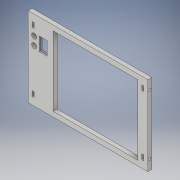
# Autodesk Inventor part: Topshelf
Saved by Autodesk Inventor 2019 (Build 230136000, 136)
## iProperties
Created: 2018-12-26
Part Number: Topshelf
Material: Generic
Document SubType Name: Modeling
Designer: Martin
Density: 1 g/cm^3
Appearance: Default
Author: Martin
Autodesk Inventor part; units mm, degrees
ref_plane "YZ Plane" through (0, 0, 0) normal (1, 0, 0) x (0, 1, 0)
ref_plane "XZ Plane" through (0, 0, 0) normal (0, 1, 0) x (-1, 0, 0)
ref_plane "XY Plane" through (0, 0, 0) normal (0, 0, 1) x (1, 0, 0)
sketch "Sketch1" plane through (0, 0, 0) normal (0, 0, 1) x (1, 0, 0)
  line L0 (-59.525, 40) -> (60.475, 40)
  line L1 (60.475, 40) -> (60.475, -40)
  line L2 (60.475, -40) -> (-59.525, -40)
  line L3 (-59.525, -40) -> (-59.525, 40)
  line L4 (-59.525, 40) -> (60.475, -40) construction
  line L5 (60.475, 40) -> (-59.525, -40) construction
  line L6 (-34.525, -65) -> (-34.525, 60.8703) construction
  line L7 (50.475, -61.0061) -> (50.475, 64.8642) construction
  line L8 (-67.2304, -35) -> (77.4738, -35) construction
  line L9 (-68.2264, 35) -> (76.4779, 35) construction
  line L10 (-2.025, -66.0646) -> (-2.025, 59.8057) construction
  line L11 (2.975, -64.9269) -> (2.975, 60.9434) construction
  line L12 (-67.6256, -30) -> (77.0786, -30) construction
  line L13 (-69.0671, 30) -> (75.6371, 30) construction
  line L14 (55.475, -60.5874) -> (55.475, 65.2829) construction
  line L15 (-54.525, -62.7211) -> (-54.525, 63.1492) construction
  line L16 (-55.475, -32.5) -> (-53.575, -32.5)
  line L17 (-53.575, -32.5) -> (-53.575, -27.5)
  line L18 (-53.575, -27.5) -> (-55.475, -27.5)
  line L19 (-55.475, -27.5) -> (-55.475, -32.5)
  line L20 (-55.475, -32.5) -> (-53.575, -27.5) construction
  line L21 (-53.575, -32.5) -> (-55.475, -27.5) construction
  line L22 (56.425, -32.5) -> (54.525, -32.5)
  line L23 (54.525, -32.5) -> (54.525, -27.5)
  line L24 (54.525, -27.5) -> (56.425, -27.5)
  line L25 (56.425, -27.5) -> (56.425, -32.5)
  line L26 (56.425, -32.5) -> (54.525, -27.5) construction
  line L27 (54.525, -32.5) -> (56.425, -27.5) construction
  line L28 (-53.575, 32.5) -> (-55.475, 32.5)
  line L29 (-55.475, 32.5) -> (-55.475, 27.5)
  line L30 (-55.475, 27.5) -> (-53.575, 27.5)
  line L31 (-53.575, 27.5) -> (-53.575, 32.5)
  line L32 (-53.575, 32.5) -> (-55.475, 27.5) construction
  line L33 (-55.475, 32.5) -> (-53.575, 27.5) construction
  line L34 (56.425, 32.5) -> (54.525, 32.5)
  line L35 (54.525, 32.5) -> (54.525, 27.5)
  line L36 (54.525, 27.5) -> (56.425, 27.5)
  line L37 (56.425, 27.5) -> (56.425, 32.5)
  line L38 (56.425, 32.5) -> (54.525, 27.5) construction
  line L39 (54.525, 32.5) -> (56.425, 27.5) construction
  line L40 (-34.525, 35) -> (50.475, 35)
  line L41 (50.475, 35) -> (50.475, -35)
  line L42 (50.475, -35) -> (-34.525, -35)
  line L43 (-34.525, -35) -> (-34.525, 35)
  point P0 (0.475, 0)
  point P1 (-2.025, 35)
  point P2 (2.975, -35)
  point P3 (50.475, 35)
  point P4 (55.475, 36)
  point P5 (56, 37)
  point P6 (-54.525, -30)
  point P7 (55.475, -30)
  point P8 (-54.525, 30)
  point P9 (55.475, 30)
  dimension "d0" = 120
  dimension "d1" = 80
  dimension "d9" = 25
  dimension "d10" = 10
  dimension "d11" = 5
  dimension "d12" = 5
  dimension "d20" = 10
  dimension "d21" = 10
  dimension "d22" = 5
  dimension "d23" = 5
  dimension "d26" = 1.9
  dimension "d27" = 5
  dimension "d28" = 1.9
  dimension "d29" = 1.9
  dimension "d30" = 5
  dimension "d31" = 1.9
  constraints: 88 end point, 23 point on line, 12 parallel, 10 horizontal, 9 midpoint, 6 perpendicular, 6 vertical
  measures "d0" distance of L1.end L2.end
  measures "d1" distance of L0.end L1.end
  measures "d9" distance between parallel lines of L6 L3
  measures "d10" distance between parallel lines of L1 L7
  measures "d11" distance between parallel lines of L8 L2
  measures "d12" distance between parallel lines of L0 L9
  measures "d20" distance between parallel lines of L12 L2
  measures "d21" distance between parallel lines of L13 L0
  measures "d22" distance between parallel lines of L14 L1
  measures "d23" distance between parallel lines of L15 L3
  measures "d26" distance of L18.end L17.end
  measures "d27" distance of L17.end L16.end
  measures "d28" distance of L23.end L24.end
  measures "d29" distance of L30.end L29.end
  measures "d30" distance of L29.end L28.end
  measures "d31" distance of L36.end L35.end
extrude "Extrusion1" add sketch "Sketch1" along normal blind 4 contours L0 L1 L2 L3 | L19 L18 L17 L16 | L22 L23 L24 L25 | L31 L30 L29 L28 | L37 L36 L35 L34 | L40 L41 L42 L43
sketch "Sketch2" plane through (60.475, -40, 0) normal (1, 0, 0) x (0, 0, -1)
  line L0 (0, 40) -> (-8.8455, 40) construction
  line L1 (-2, -5.0193) -> (-2, 56.2537) construction
  line L2 (-4, 0) -> (-4, 80) construction
  line L3 (1.2244, 10) -> (-7.6211, 10) construction
  line L4 (0, 0) -> (-4, 0) construction
  circle A0 centre (-2, 10) radius 1.25
  circle A1 centre (-2, 70) radius 1.25
  dimension "d4" = 2
  dimension "d5" = 10
  dimension "d6" = 2.5
  constraints: 6 end point, 2 centre point, 2 horizontal, 2 point on line, 1 symmetric about line, 1 vertical, 1 other
  measures "d4" distance between parallel lines of L1 L2
  measures "d5" distance between parallel lines of L3 L4
  measures "d6" diameter of A0
extrude "Extrusion3" cut sketch "Sketch2" against normal blind 10
extrude "Extrusion4" cut sketch "Sketch1" along normal blind 10 contours L19 L18 L17 L16 | L22 L23 L24 L25 | L31 L30 L29 L28 | L37 L36 L35 L34
ref_plane "Work Plane1" through (0.475, -40, 0) normal (1, 0, 0) x (0, 0, -1)
mirror "Mirror1" about plane through (0.475, -40, 0) normal (1, 0, 0) of "Extrusion3"
extrude "Extrusion6" cut sketch "Sketch1" along normal blind 10 contours L40 L41 L42 L43
sketch "Sketch3" plane through (0, 0, 4) normal (0, 0, 1) x (1, 0, 0)
  line L0 (0, 0) -> (-78.4813, 0) construction
  line L1 (-44.525, 48.1643) -> (-44.525, -53.6198) construction
  line L2 (-34.525, -35) -> (-34.525, 35) construction
  line L3 (-48.525, 23.5) -> (-40.525, 23.5)
  line L4 (-40.525, 23.5) -> (-40.525, 10)
  line L5 (-40.525, 10) -> (-48.525, 10)
  line L6 (-48.525, 10) -> (-48.525, 23.5)
  line L7 (-53.525, 48.2216) -> (-53.525, -53.5625) construction
  circle A0 centre (-53.525, 20.95) radius 2.55
  circle A1 centre (-53.525, 12.55) radius 2.55
  line L8 (-47.3423, 23.5) -> (-70.4402, 23.5) construction
  line L9 (-47.3423, 10) -> (-69.2245, 10) construction
  line L10 (60.475, 40) -> (-59.525, 40) projected
  point P0 (-44.525, 0)
  point P1 (-53.525, 1)
  dimension "d38" = 10
  dimension "d39" = 8
  dimension "d40" = 13.5
  dimension "d41" = 5
  dimension "d42" = 5.1
  dimension "d43" = 5.1
  dimension "d47" = 30
  constraints: 18 end point, 8 point on line, 3 horizontal, 2 centre point, 2 parallel, 2 tangent, 2 vertical, 1 perpendicular
  measures "d38" distance between parallel lines of L1 L2
  measures "d39" distance of L4.end L5.end
  measures "d40" distance of L3.end L4.end
  measures "d41" distance between parallel lines of L7 L6
  measures "d42" diameter of A0
  measures "d43" diameter of A1
  measures "d47" distance between parallel lines of L9 L10
extrude "Extrusion7" cut sketch "Sketch3" against normal blind 10
sketch "Sketch5" plane through (0, 0, 0) normal (0, 0, -1) x (-1, 0, 0)
  line L0 (48.525, 10) -> (40.525, 10) construction
  line L1 (40.525, 10) -> (40.525, 23.5) construction
  line L2 (40.525, 23.5) -> (48.525, 23.5) construction
  line L3 (48.525, 23.5) -> (48.525, 10) construction
  line L4 (48.525, 10) -> (40.525, 10) construction
  line L5 (48.525, 23.5) -> (48.525, 10) construction
  line L6 (49.525, 9) -> (39.525, 9)
  line L7 (39.525, 9) -> (39.525, 24.5)
  line L8 (39.525, 24.5) -> (49.525, 24.5)
  line L9 (49.525, 24.5) -> (49.525, 9)
  point P0 (0, 0)
  dimension "d48" = 1
  constraints: 16 end point, 4 parallel, 2 collinear, 2 perpendicular, 1 horizontal, 3 other
  measures "d48" distance between parallel lines of L3 L9
extrude "Extrusion8" cut sketch "Sketch5" against normal blind 3
body "Solid1"
